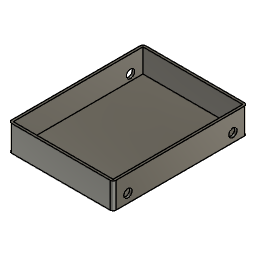
rc (1) (Autodesk Fusion 360 design; units mm, degrees)
Autodesk Fusion 360 part; units mm, degrees
sketch "Sketch1" plane through (0, 0, 0) normal (0, 0, 1) x (1, 0, 0)
  line L0 (0, 0) -> (177.8, 0)
  line L1 (177.8, 0) -> (177.8, 228.6)
  line L2 (177.8, 228.6) -> (0, 228.6)
  line L3 (0, 228.6) -> (0, 0)
  dimension "d1" = 177.8
  dimension "d2" = 228.6
  constraint horizontal L0
  constraint vertical L1
  constraint horizontal L2
  constraint vertical L3
  constraint coincident L0.start L3.end
  measures "d1" distance of L0.start L0.end
  measures "d2" distance of L0.start L2.end
extrude "Extrude1" add sketch "Sketch1" along normal blind 4
extrude "Extrude2" add 1 faces at (59.2667, 152.4, 4) along direction (0, 0, 1) blind 40 thin wall 4 inside
hole "Hole1" at (177.8, 25.2182, 14.7531) direction (-1, 0, 0) diameter 14 depth 15 tip angle 118
hole "Hole2" at (177.8, 204.0495, 14.6495) direction (-1, 0, 0) diameter 14 depth 15 tip angle 118
hole "Hole3" at (0, 203.4824, 14.8106) direction (1, 0, 0) diameter 14 depth 15 tip angle 118
hole "Hole4" at (0, 23.8632, 14.9096) direction (1, 0, 0) diameter 14 depth 15 tip angle 118
fillet "Fillet1" radius 5 1 edges at (0, 0, 22)
fillet "Fillet2" radius 5 1 edges at (177.8, 0, 22)
fillet "Fillet3" radius 5 1 edges at (177.8, 228.6, 22)
fillet "Fillet4" radius 5 1 edges at (0, 228.6, 22)
